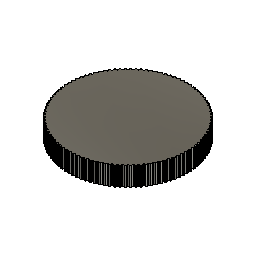
gear_100z (Autodesk Fusion 360 design; units mm, degrees)
Autodesk Fusion 360 part; units mm, degrees
sketch "Sketch1" plane through (0, 0, 0) normal (0, 0, 1) x (1, 0, 0) in component "gt2 pulley"
  circle A0 centre (0, 0) radius 31.831 construction
  circle A1 centre (0, 0) radius 30.827 construction
  line L0 (0, 0) -> (0, 31.831) construction
  line L1 (0, 0) -> (0.9998, 31.8153) construction
  line L2 (0, 0) -> (1.404, 31.8) construction
  circle A2 centre (0, 0) radius 31.577 construction
  arc A3 (0.3983, 31.4417) -> (0.478, 31.1423) centre (1.3928, 31.5463) ccw
  circle A4 centre (0, 0) radius 31.427 construction
  arc A5 (0.2502, 31.576) -> (0, 31.577) centre (0, 0) ccw
  arc A6 (0.3983, 31.4417) -> (0.2502, 31.576) centre (0.2491, 31.426) ccw
  arc A7 (0.478, 31.1423) -> (0.9683, 30.8118) centre (0.9857, 31.3665) ccw
  arc A8 (0, 31.577) -> (-0.2502, 31.576) centre (0, 0) ccw
  arc A9 (-0.2502, 31.576) -> (-0.3983, 31.4417) centre (-0.2491, 31.426) ccw
  arc A10 (-0.478, 31.1423) -> (-0.3983, 31.4417) centre (-1.3928, 31.5463) ccw
  arc A11 (-0.9684, 30.8118) -> (-0.478, 31.1423) centre (-0.9857, 31.3665) ccw
  arc A12 (0.9683, 30.8118) -> (-0.9683, 30.8118) centre (0, 0) ccw
  point P0 (1.3928, 31.5463)
  point P1 (0, 31.577)
  dimension "d18" = 63.662
  dimension "d19" = 1.8
  dimension "d22" = 1.004
  dimension "d24" = 0.75
  dimension "d26" = 1
  dimension "d27" = 0.15
  dimension "d28" = 0.15
  dimension "d47" = 0.555
  dimension "d52" = 3.812
  constraint coincident A0.centre A1.centre
  constraint coincident A0 L0.end
  constraint vertical L0
  constraint coincident A0 L1.end
  constraint coincident A0 L2.end
  constraint concentric A1 A2
  constraint coincident A1 A7.end
  constraint coincident L1 A7.end
  constraint coincident A2 P0
  constraint coincident L2 P0
  constraint coincident P0 A3.centre
  constraint coincident A2 P1
  constraint coincident L0 P1
  constraint concentric A2 A4
  constraint coincident P1 A5.end
  constraint coincident A4 A6.centre
  constraint coincident A3.start A6.start
  constraint tangent A3 A6
  constraint tangent A3 A7
  constraint symmetric L0 A7.end A12.end
  constraint symmetric L0 A3.start A9.end
  constraint symmetric L0 A3.end A10.start
  constraint symmetric L0 A3 A10
  constraint symmetric L0 A5.start A8.end
  constraint symmetric L0 P1 A5.end
  constraint symmetric L0 A5 A8
  constraint symmetric L0 A6 A9
  constraint symmetric L0 A7 A11
  constraint coincident A1 A11.start
  constraint tangent A1 A7
  constraint coincident L1 A7.centre
  measures "d18" diameter of A0
  measures "d19" angle of L0 L1
  measures "d22" distance of A0 A1
  measures "d24" distance of A1 A2
  measures "d26" radius of A3
  measures "d27" distance of A2 A4
  measures "d28" radius of A6
  measures "d47" radius of A7
extrude "Extrude1" add sketch "Sketch1" along normal blind 10 makes body 1
pattern_circular "C-Pattern1" count 100 over 360 about axis through (0, 0, 1.75) along (0, 0, 1) of bodies 1 makes body 2 at (-2.6869, 30.7097, 6.6667) makes body 3 at (-3.9704, 30.5702, 6.6667) makes body 4 at (-5.0349, 30.413, 3.3333) makes body 5 at (-8.3937, 29.6623, 6.6667) makes body 6 at (-8.8069, 29.5422, 3.3333) makes body 7 at (-12.0452, 28.3764, 6.6667) makes body 8 at (-13.2228, 27.8471, 6.6667) makes body 9 at (-14.9453, 26.9619, 6.6667) makes body 10 at (-15.8771, 26.4239, 3.3333) makes body 11 at (-18.2066, 24.8761, 6.6667) makes body 12 at (-19.0637, 24.2256, 3.3333) makes body 13 at (-21.1809, 22.3981, 6.6667) makes body 14 at (-21.9496, 21.6453, 6.6667) makes body 15 at (-24.2257, 19.0636, 6.6667) makes body 16 at (-24.4894, 18.7236, 3.3333) makes body 17 at (-25.6168, 17.1489, 3.3333) makes body 18 at (-27.3687, 14.1865, 6.6667) makes body 19 at (-27.5641, 13.8031, 3.3333) makes body 20 at (-28.7017, 11.248, 6.6667) makes body 21 at (-29.0767, 10.2395, 3.3333) makes body 22 at (-29.6623, 8.3936, 3.3333) makes body 23 at (-30.3009, 5.6706, 6.6667) makes body 24 at (-30.6692, 3.1152, 6.6667) makes body 25 at (-30.8043, 1.1833, 6.6667) makes body 26 at (-30.8178, -0.7533, 6.6667) makes body 27 at (-30.7097, -2.6869, 6.6667) makes body 28 at (-30.5702, -3.9704, 6.6667) makes body 29 at (-30.413, -5.0349, 3.3333) makes body 30 at (-29.6623, -8.3937, 6.6667) makes body 31 at (-29.5422, -8.8069, 3.3333) makes body 32 at (-28.3764, -12.0452, 6.6667) makes body 33 at (-27.564, -13.8032, 6.6667) makes body 34 at (-27.3687, -14.1866, 3.3333) makes body 35 at (-26.4239, -15.8771, 3.3333) makes body 36 at (-24.4893, -18.7237, 6.6667) makes body 37 at (-24.2256, -19.0637, 3.3333) makes body 38 at (-22.9808, -20.5472, 6.6667) makes body 39 at (-20.7071, -22.8368, 6.6667) makes body 40 at (-19.5668, -23.8211, 6.6667) makes body 41 at (-18.7236, -24.4894, 3.3333) makes body 42 at (-17.1489, -25.6168, 3.3333) makes body 43 at (-14.1865, -27.3687, 6.6667) makes body 44 at (-13.8031, -27.5641, 3.3333) makes body 45 at (-10.6444, -28.931, 6.6667) makes body 46 at (-10.2395, -29.0767, 3.3333) makes body 47 at (-8.3936, -29.6623, 3.3333) makes body 48 at (-6.5145, -30.1308, 3.3333) makes body 49 at (-3.7568, -30.5972, 6.6667) makes body 50 at (-2.6867, -30.7097, 3.3333) makes body 51 at (0.7533, -30.8178, 6.6667) makes body 52 at (2.6869, -30.7097, 6.6667) makes body 53 at (3.9704, -30.5702, 6.6667) makes body 54 at (5.8821, -30.2606, 6.6667) makes body 55 at (8.3937, -29.6623, 6.6667) makes body 56 at (8.8069, -29.5422, 3.3333) makes body 57 at (12.0452, -28.3764, 6.6667) makes body 58 at (13.2228, -27.8471, 6.6667) makes body 59 at (14.9453, -26.9619, 6.6667) makes body 60 at (15.8771, -26.4239, 3.3333) makes body 61 at (18.7237, -24.4893, 6.6667) makes body 62 at (19.0637, -24.2256, 6.6667) makes body 63 at (21.1809, -22.3981, 6.6667) makes body 64 at (21.9496, -21.6453, 6.6667) makes body 65 at (23.8211, -19.5668, 6.6667) makes body 66 at (24.4894, -18.7236, 3.3333) makes body 67 at (26.4239, -15.877, 6.6667) makes body 68 at (27.3687, -14.1865, 6.6667) makes body 69 at (27.5641, -13.8031, 3.3333) makes body 70 at (28.7017, -11.248, 6.6667) makes body 71 at (29.0767, -10.2395, 3.3333) makes body 72 at (29.6623, -8.3936, 3.3333) makes body 73 at (30.1308, -6.5145, 3.3333) makes body 74 at (30.5972, -3.7568, 6.6667) makes body 75 at (30.8043, -1.1833, 6.6667) makes body 76 at (30.8178, 0.7533, 6.6667) makes body 77 at (30.7097, 2.6869, 6.6667) makes body 78 at (30.5702, 3.9704, 6.6667) makes body 79 at (30.1308, 6.5146, 6.6667) makes body 80 at (29.6623, 8.3937, 6.6667) makes body 81 at (29.5422, 8.8069, 3.3333) makes body 82 at (28.3764, 12.0452, 6.6667) makes body 83 at (27.8471, 13.2228, 6.6667) makes body 84 at (26.9619, 14.9453, 6.6667) makes body 85 at (26.4239, 15.8771, 3.3333) makes body 86 at (24.8761, 18.2066, 6.6667) makes body 87 at (24.2256, 19.0637, 6.6667) makes body 88 at (22.3981, 21.1809, 6.6667) makes body 89 at (20.7071, 22.8368, 6.6667) makes body 90 at (19.5668, 23.8211, 6.6667) makes body 91 at (18.7236, 24.4894, 3.3333) makes body 92 at (15.877, 26.4239, 6.6667) makes body 93 at (14.1865, 27.3687, 6.6667) makes body 94 at (13.8031, 27.5641, 3.3333) makes body 95 at (11.248, 28.7017, 6.6667) makes body 96 at (10.2395, 29.0767, 3.3333) makes body 97 at (8.3936, 29.6623, 3.3333) makes body 98 at (6.5145, 30.1308, 3.3333) makes body 99 at (3.1152, 30.6692, 6.6667) makes body 100 at (2.6867, 30.7097, 3.3333)
sketch "Sketch2" plane through (0, 0, 10) normal (0, 0, 1) x (-1, 0, 0)
  arc A0 (-15.4962, -27.3607) -> (-15.4311, -27.5497) centre (-15.3579, -27.4188) ccw
  arc A1 (-15.4311, -27.5497) -> (-14.9926, -27.7908) centre (0, 0) ccw
  arc A2 (-14.9926, -27.7908) -> (-14.7981, -27.7444) centre (-14.9213, -27.6588) ccw
  arc A3 (-14.584, -27.5205) -> (-14.7981, -27.7444) centre (-13.977, -28.3152) ccw
  arc A4 (-13.9952, -27.467) -> (-14.584, -27.5205) centre (-14.2471, -27.9616) ccw
  arc A5 (-15.6922, -26.5341) -> (-13.9952, -27.467) centre (0, 0) ccw
  arc A6 (-15.4218, -27.0599) -> (-15.6922, -26.5341) centre (-15.9747, -27.0118) ccw
  arc A7 (-15.4962, -27.3607) -> (-15.4218, -27.0599) centre (-16.4181, -26.9732) ccw
  circle A8 centre (0, 0) radius 30.827
  constraint coincident A1.centre A5.centre
extrude "Extrude2" add sketch "Sketch2" against normal blind 10 contours A5 A8 bodies 1 2 3 4 5 6 7 8 9 10 11 12 13 14 15 16 17 18 19 20 21 22 23 24 25 26 27 28 29 30 31 32 33 34 35 36 37 38 39 40 41 42 43 44 45 46 47 48 49 50 51 52 53 54 55 56 57 58 59 60 61 62 63 64 65 66 67 68 69 70 71 72 73 74 75 76 77 78 79 80 81 82 83 84 85 86 87 88 89 90 91 92 93 94 95 96 97 98 99 100
extrude "Extrude4" [suppressed] in component "gt2 pulley"
pattern_circular "C-Pattern7" [suppressed] in component "gt2 pulley"
extrude "Extrude3" [suppressed] in component "gt2 pulley"
pattern_circular "C-Pattern6" [suppressed] in component "gt2 pulley"
extrude "Extrude2'" [suppressed] in component "gt2 pulley"
pattern_circular "C-Pattern5" [suppressed] in component "gt2 pulley"
extrude "Extrude1'" [suppressed] in component "gt2 pulley"
pattern_circular "C-Pattern4" [suppressed] in component "gt2 pulley"
pattern_circular "C-Pattern3" [suppressed] in component "gt2 pulley"
pattern_circular "C-Pattern2" [suppressed] in component "gt2 pulley"
pattern_circular "C-Pattern1'" [suppressed] in component "gt2 pulley"
copy_body "Body->Comp1" [suppressed] in component "Component"
copy_body "Body->Comp2" [suppressed] in component "Component'"
copy_body "Body->Comp3" [suppressed] in component "Component''"
copy_body "Body->Comp4" [suppressed] in component "Component'''"
copy_body "Body->Comp5" [suppressed] in component "Component''''"
copy_body "Body->Comp6" [suppressed] in component "Component'''''"
copy_body "Body->Comp7" [suppressed] in component "Component''''''"
copy_body "Body->Comp8" [suppressed] in component "Component'''''''"
copy_body "Body->Comp9" [suppressed] in component "Component''''''''"
copy_body "Body->Comp10" [suppressed] in component "Component'''''''''"
copy_body "Body->Comp11" [suppressed] in component "Component''''''''''"
copy_body "Body->Comp12" [suppressed] in component "Component'''''''''''"
copy_body "Body->Comp13" [suppressed] in component "Component''''''''''''"
copy_body "Body->Comp14" [suppressed] in component "Component'''''''''''''"
copy_body "Body->Comp15" [suppressed] in component "Component''''''''''''''"
copy_body "Body->Comp16" [suppressed] in component "Component'''''''''''''''"
copy_body "Body->Comp17" [suppressed] in component "Component''''''''''''''''"
copy_body "Body->Comp18" [suppressed] in component "Component'''''''''''''''''"
copy_body "Body->Comp19" [suppressed] in component "Component''''''''''''''''''"
copy_body "Body->Comp20" [suppressed] in component "Component'''''''''''''''''''"
component "gt2 pulley" placed x (1, 0, 0) y (0, 1, 0) z (0, 0, 1) at (0, 0, 0)
equation "NumTeeth = 100" comment "min 20"
equation "ToothPitch = 2 mm"
equation "PullyDia = NumTeeth * ToothPitch / PI"
equation "ToothAng = ( ( 360 / NumTeeth ) * 1 deg )"
equation "TransOffsetAngle = ToothAng * 0.2"
equation "Sholulder_Radius = 0.15 mm"
equation "Root_Radius = 0.555 mm"
equation "TransRadius = 1 mm"
equation "ToolHeight = 0.75 mm"
equation "PLD = 0.254 mm"
equation "d18 = PullyDia"
equation "d19 = ToothAng / 2"
equation "d22 = PLD + ToolHeight"
equation "d24 = ToolHeight"
equation "d26 = TransRadius"
equation "d27 = Sholulder_Radius"
equation "d31 = NumTeeth"
equation "d33 = NumTeeth"
equation "d35 = NumTeeth"
equation "d37 = NumTeeth"
equation "d41 = NumTeeth"
equation "d45 = NumTeeth"
equation "d47 = Root_Radius"
equation "d50 = NumTeeth"
